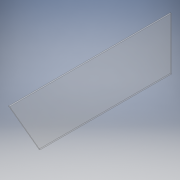
# Autodesk Inventor part: PaddleCollection2.1Casing
Saved by Autodesk Inventor 2019 (Build 230136000, 136)
## iProperties
Created: 2018-10-20
Part Number: PaddleCollection2.1Casing
Material: Polycarbonate, Clear
Document SubType Name: Modeling
Designer: User
Density: 1.2 g/cm^3
Appearance: Polycarbonate - Clear
Mass: 36.0285 g
Surface Area: 334.77 cm^2
Volume: 30.0237 cm^3
Author: User
Autodesk Inventor part; units mm, degrees
ref_plane "YZ Plane" through (0, 0, 0) normal (1, 0, 0) x (0, 1, 0)
ref_plane "XZ Plane" through (0, 0, 0) normal (0, 1, 0) x (-1, 0, 0)
ref_plane "XY Plane" through (0, 0, 0) normal (0, 0, 1) x (1, 0, 0)
sketch "Sketch1" plane through (0, 0, 0) normal (1, 0, 0) x (0, 1, 0)
  line L0 (0, 0) -> (76.2, 0)
  line L1 (76.2, 0) -> (76.2, -234.4941)
  line L2 (76.2, -234.4941) -> (0, -234.4941)
  line L3 (0, -234.4941) -> (0, 0)
  line L4 (76.2, 0) -> (0, -43.9941)
  line L5 (76.2, 0) -> (164.1882, 0) construction
  dimension "d0" = 76.2
  dimension "d2" = 150
  dimension "d5" = 190.5
  constraints: 12 end point, 2 horizontal, 2 parallel, 1 equal length, 1 perpendicular, 1 point on line
  measures "d0" distance of L1.end L2.end
  measures "d2" angle of L4 L5
  measures "d5" distance from line of L2 L4.end
extrude "Extrusion1" add sketch "Sketch1" along normal blind 1.8542 contours L1 L2 L3 L4
body "Solid1"
